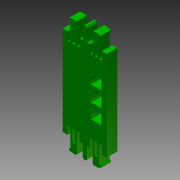
# Autodesk Inventor part: floor_front
Saved by Autodesk Inventor 2012 SP1 (Build 160190100, 190)
## iProperties
Created: 2011-10-14
Part Number: floor_front
Document SubType Name: Modeling
Designer: cramera
Density: 0.952 g/cm^3
Material: High Density Polyethylene
Mass: 57.2272 g
Surface Area: 209.441 cm^2
Volume: 60.1126 cm^3
Autodesk Inventor part; units mm, degrees
ref_plane "YZ Plane" through (0, 0, 0) normal (1, 0, 0) x (0, 1, 0)
ref_plane "XZ Plane" through (0, 0, 0) normal (0, 1, 0) x (-1, 0, 0)
ref_plane "XY Plane" through (0, 0, 0) normal (0, 0, 1) x (1, 0, 0)
derived "skeleton.ipt"
sketch "STOCK_12MM" plane through (0, 0, 0) normal (0, 0, 1) x (1, 0, 0)
  line L0 (457.2, 914.4) -> (457.2, 0)
  line L1 (0, 0) -> (457.2, 0)
  line L2 (457.2, 0) -> (457.2, 914.4)
  line L3 (457.2, 914.4) -> (0, 914.4)
  line L4 (0, 914.4) -> (0, 0)
  constraints: 10 end point
sketch "THROUGH-CUT" plane through (0, 0, 0) normal (0, 0, 1) x (1, 0, 0)
  arc A0 (302.181, 142.2396) -> (299.936, 144.4847) centre (301.0585, 143.3622) ccw
  line L0 (302.181, 142.2396) -> (302.181, 136.5697)
  arc A1 (299.936, 134.3247) -> (302.181, 136.5697) centre (301.0585, 135.4472) ccw
  line L1 (299.936, 134.3247) -> (292.1071, 134.3247)
  arc A2 (289.862, 136.5697) -> (292.1071, 134.3247) centre (290.9846, 135.4472) ccw
  line L2 (289.862, 136.5697) -> (289.862, 142.2396)
  arc A3 (292.1071, 144.4847) -> (289.862, 142.2396) centre (290.9846, 143.3622) ccw
  line L3 (292.1071, 144.4847) -> (299.936, 144.4847)
  line L4 (292.1071, 116.4177) -> (299.936, 116.4177)
  arc A4 (299.936, 116.4177) -> (302.181, 118.6627) centre (301.0585, 117.5402) ccw
  line L5 (302.181, 118.6627) -> (302.181, 125.6026)
  arc A5 (302.181, 125.6026) -> (299.936, 127.8477) centre (301.0585, 126.7252) ccw
  line L6 (299.936, 127.8477) -> (292.1071, 127.8477)
  arc A6 (292.1071, 127.8477) -> (289.862, 125.6026) centre (290.9846, 126.7252) ccw
  line L7 (289.862, 125.6026) -> (289.862, 118.6627)
  arc A7 (289.862, 118.6627) -> (292.1071, 116.4177) centre (290.9846, 117.5402) ccw
  line L8 (292.1071, 99.7807) -> (299.936, 99.7807)
  arc A8 (299.936, 99.7807) -> (302.181, 102.0257) centre (301.0585, 100.9032) ccw
  line L9 (302.181, 102.0257) -> (302.181, 107.6956)
  arc A9 (302.181, 107.6956) -> (299.936, 109.9407) centre (301.0585, 108.8182) ccw
  line L10 (299.936, 109.9407) -> (292.1071, 109.9407)
  arc A10 (292.1071, 109.9407) -> (289.862, 107.6956) centre (290.9846, 108.8182) ccw
  line L11 (289.862, 107.6956) -> (289.862, 102.0257)
  arc A11 (289.862, 102.0257) -> (292.1071, 99.7807) centre (290.9846, 100.9032) ccw
  arc A12 (270.3675, 164.2014) -> (271.955, 165.7889) centre (270.3675, 165.7889) ccw
  line L12 (271.955, 165.7889) -> (271.955, 177.3174)
  arc A13 (271.955, 177.3174) -> (270.3675, 178.9049) centre (270.3675, 177.3174) ccw
  line L13 (270.3675, 178.9049) -> (270.2405, 178.9049)
  arc A14 (270.2405, 178.9049) -> (268.653, 177.3174) centre (270.2405, 177.3174) ccw
  line L14 (268.653, 177.3174) -> (268.653, 165.7889)
  arc A15 (268.653, 165.7889) -> (270.2405, 164.2014) centre (270.2405, 165.7889) ccw
  line L15 (270.2405, 164.2014) -> (270.3675, 164.2014)
  arc A16 (295.8945, 178.9049) -> (294.307, 177.3174) centre (295.8945, 177.3174) ccw
  line L16 (295.8945, 178.9049) -> (296.0215, 178.9049)
  arc A17 (297.609, 177.3174) -> (296.0215, 178.9049) centre (296.0215, 177.3174) ccw
  line L17 (297.609, 177.3174) -> (297.609, 165.7889)
  arc A18 (296.0215, 164.2014) -> (297.609, 165.7889) centre (296.0215, 165.7889) ccw
  line L18 (296.0215, 164.2014) -> (295.8945, 164.2014)
  arc A19 (294.307, 165.7889) -> (295.8945, 164.2014) centre (295.8945, 165.7889) ccw
  line L19 (294.307, 165.7889) -> (294.307, 177.3174)
  arc A20 (271.955, 78.4764) -> (270.3675, 80.0639) centre (270.3675, 78.4764) ccw
  line L20 (271.955, 78.4764) -> (271.955, 66.948)
  arc A21 (270.3675, 65.3605) -> (271.955, 66.948) centre (270.3675, 66.948) ccw
  line L21 (270.3675, 65.3605) -> (270.2405, 65.3605)
  arc A22 (268.653, 66.948) -> (270.2405, 65.3605) centre (270.2405, 66.948) ccw
  line L22 (268.653, 66.948) -> (268.653, 78.4764)
  arc A23 (270.2405, 80.0639) -> (268.653, 78.4764) centre (270.2405, 78.4764) ccw
  line L23 (270.2405, 80.0639) -> (270.3675, 80.0639)
  line L24 (280.591, 56.8864) -> (280.591, 68.2939)
  arc A24 (280.591, 68.2939) -> (278.346, 70.5389) centre (279.4685, 69.4164) ccw
  line L25 (278.346, 70.5389) -> (277.289, 70.5389)
  line L26 (277.289, 70.5389) -> (277.289, 78.4764)
  arc A25 (277.289, 78.4764) -> (275.7015, 80.0639) centre (275.7015, 78.4764) ccw
  line L27 (275.7015, 80.0639) -> (275.5745, 80.0639)
  arc A26 (275.5745, 80.0639) -> (273.987, 78.4764) centre (275.5745, 78.4764) ccw
  line L28 (273.987, 78.4764) -> (273.987, 56.8864)
  arc A27 (272.4017, 55.2989) -> (273.987, 56.8864) centre (272.3995, 56.8864) ccw
  line L29 (272.4017, 55.2989) -> (268.6966, 55.2989)
  line L30 (268.6966, 55.2989) -> (265.097, 56.121)
  line L31 (265.097, 56.121) -> (265.097, 57.8389)
  line L32 (265.097, 57.8389) -> (266.621, 59.1089)
  line L33 (266.621, 59.1089) -> (266.621, 61.7362)
  line L34 (266.621, 61.7362) -> (266.621, 78.4764)
  arc A28 (266.621, 78.4764) -> (265.0335, 80.0639) centre (265.0335, 78.4764) ccw
  line L35 (265.0335, 80.0639) -> (264.9065, 80.0639)
  arc A29 (264.9065, 80.0639) -> (263.319, 78.4764) centre (264.9065, 78.4764) ccw
  line L36 (263.319, 78.4764) -> (263.319, 70.5389)
  line L37 (263.319, 70.5389) -> (257.731, 70.5389)
  line L38 (257.731, 70.5389) -> (257.731, 173.7264)
  line L39 (257.731, 173.7264) -> (263.319, 173.7264)
  line L40 (263.319, 173.7264) -> (263.319, 165.7889)
  arc A30 (263.319, 165.7889) -> (264.9065, 164.2014) centre (264.9065, 165.7889) ccw
  line L41 (264.9065, 164.2014) -> (265.0335, 164.2014)
  arc A31 (265.0335, 164.2014) -> (266.621, 165.7889) centre (265.0335, 165.7889) ccw
  line L42 (266.621, 165.7889) -> (266.621, 182.5292)
  line L43 (266.621, 182.5292) -> (266.621, 185.1564)
  line L44 (266.621, 185.1564) -> (265.097, 186.4264)
  line L45 (265.097, 186.4264) -> (265.097, 188.1444)
  line L46 (265.097, 188.1444) -> (268.6966, 188.9664)
  line L47 (268.6966, 188.9664) -> (272.4017, 188.9664)
  arc A32 (273.987, 187.3789) -> (272.4017, 188.9664) centre (272.3995, 187.3789) ccw
  line L48 (273.987, 187.3789) -> (273.987, 165.7889)
  arc A33 (273.987, 165.7889) -> (275.5745, 164.2014) centre (275.5745, 165.7889) ccw
  line L49 (275.5745, 164.2014) -> (275.7015, 164.2014)
  arc A34 (275.7015, 164.2014) -> (277.289, 165.7889) centre (275.7015, 165.7889) ccw
  line L50 (277.289, 165.7889) -> (277.289, 173.7264)
  line L51 (277.289, 173.7264) -> (278.346, 173.7264)
  arc A35 (278.346, 173.7264) -> (280.591, 175.9715) centre (279.4685, 174.849) ccw
  line L52 (280.591, 175.9715) -> (280.591, 187.3789)
  line L53 (280.591, 187.3789) -> (282.1785, 188.9664)
  line L54 (282.1785, 188.9664) -> (284.0835, 188.9664)
  line L55 (284.0835, 188.9664) -> (285.671, 187.3789)
  line L56 (285.671, 187.3789) -> (285.671, 175.9715)
  arc A36 (285.671, 175.9715) -> (285.671, 173.7264) centre (286.7936, 174.849) ccw
  arc A37 (285.671, 173.7264) -> (287.9161, 173.7264) centre (286.7936, 174.849) ccw
  line L57 (287.9161, 173.7264) -> (288.973, 173.7264)
  line L58 (288.973, 173.7264) -> (288.973, 165.7889)
  arc A38 (288.973, 165.7889) -> (290.5605, 164.2014) centre (290.5605, 165.7889) ccw
  line L59 (290.5605, 164.2014) -> (290.6875, 164.2014)
  arc A39 (290.6875, 164.2014) -> (292.275, 165.7889) centre (290.6875, 165.7889) ccw
  line L60 (292.275, 165.7889) -> (292.275, 187.3789)
  arc A40 (293.8625, 188.9664) -> (292.275, 187.3789) centre (293.8625, 187.3789) ccw
  line L61 (293.8625, 188.9664) -> (297.5655, 188.9664)
  line L62 (297.5655, 188.9664) -> (301.165, 188.1444)
  line L63 (301.165, 188.1444) -> (301.165, 186.4264)
  line L64 (301.165, 186.4264) -> (299.641, 185.1564)
  line L65 (299.641, 185.1564) -> (299.641, 182.5292)
  line L66 (299.641, 182.5292) -> (299.641, 165.7889)
  arc A41 (299.641, 165.7889) -> (301.2285, 164.2014) centre (301.2285, 165.7889) ccw
  line L67 (301.2285, 164.2014) -> (301.3555, 164.2014)
  arc A42 (301.3555, 164.2014) -> (302.943, 165.7889) centre (301.3555, 165.7889) ccw
  line L68 (302.943, 165.7889) -> (302.943, 173.7264)
  line L69 (302.943, 173.7264) -> (308.531, 173.7264)
  line L70 (308.531, 173.7264) -> (308.531, 70.5389)
  line L71 (308.531, 70.5389) -> (302.943, 70.5389)
  line L72 (302.943, 70.5389) -> (302.943, 78.4764)
  arc A43 (302.943, 78.4764) -> (301.3555, 80.0639) centre (301.3555, 78.4764) ccw
  line L73 (301.3555, 80.0639) -> (301.2285, 80.0639)
  arc A44 (301.2285, 80.0639) -> (299.641, 78.4764) centre (301.2285, 78.4764) ccw
  line L74 (299.641, 78.4764) -> (299.641, 61.7362)
  line L75 (299.641, 61.7362) -> (299.641, 59.1089)
  line L76 (299.641, 59.1089) -> (301.165, 57.8389)
  line L77 (301.165, 57.8389) -> (301.165, 56.121)
  line L78 (301.165, 56.121) -> (297.5655, 55.2989)
  line L79 (297.5655, 55.2989) -> (293.8625, 55.2989)
  arc A45 (292.275, 56.8864) -> (293.8625, 55.2989) centre (293.8625, 56.8864) ccw
  line L80 (292.275, 56.8864) -> (292.275, 78.4764)
  arc A46 (292.275, 78.4764) -> (290.6831, 80.0639) centre (290.6875, 78.4764) ccw
  line L81 (290.6831, 80.0639) -> (290.5605, 80.0639)
  arc A47 (290.5605, 80.0639) -> (288.973, 78.4764) centre (290.5605, 78.4764) ccw
  line L82 (288.973, 78.4764) -> (288.973, 70.5389)
  line L83 (288.973, 70.5389) -> (287.9161, 70.5389)
  arc A48 (287.9161, 70.5389) -> (285.671, 68.2939) centre (286.7936, 69.4164) ccw
  line L84 (285.671, 68.2939) -> (285.671, 56.8864)
  line L85 (285.671, 56.8864) -> (284.0835, 55.2989)
  line L86 (284.0835, 55.2989) -> (282.1785, 55.2989)
  line L87 (282.1785, 55.2989) -> (280.591, 56.8864)
  arc A49 (297.609, 78.4697) -> (296.0215, 80.0572) centre (296.0215, 78.4697) ccw
  line L88 (296.0215, 80.0572) -> (295.8945, 80.0639)
  arc A50 (295.8945, 80.0639) -> (294.307, 78.4764) centre (295.8945, 78.4764) ccw
  line L89 (294.307, 78.4764) -> (294.307, 66.948)
  arc A51 (294.307, 66.948) -> (295.8945, 65.3605) centre (295.8945, 66.948) ccw
  line L90 (295.8945, 65.3605) -> (296.0215, 65.3605)
  arc A52 (296.0215, 65.3605) -> (297.609, 66.948) centre (296.0215, 66.948) ccw
  line L91 (297.609, 66.948) -> (297.609, 78.4697)
  constraints: 184 end point, 106 point on circle, 53 centre point
extrude "Extrusion1" add sketch "THROUGH-CUT" along normal blind 12
equation "\"d1\" = StockThickness"
equation "\"StockThickness\" = 12"
body "Solid1"
